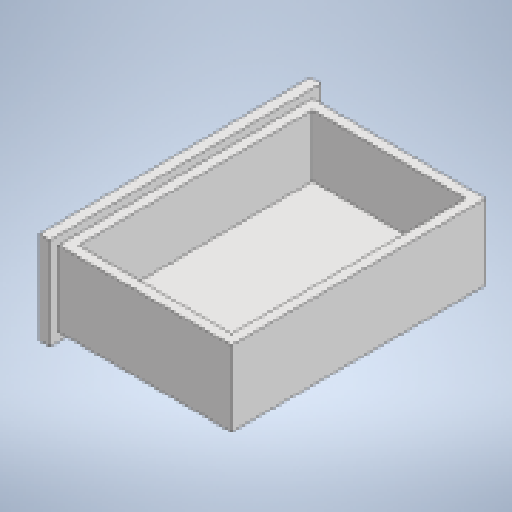
# Autodesk Inventor part: Cajon
Saved by Autodesk Inventor 2024 (Build 280153000, 153)
## iProperties
Created: 2025-02-23
Part Number: Cajon
Material: Genérico
Document SubType Name: Modeling
Designer: sergi
Density: 1 g/cm^3
Appearance: Valor por defecto
Author: sergi
Autodesk Inventor part; units mm, degrees
ref_plane "YZ Plane" through (0, 0, 0) normal (1, 0, 0) x (0, 1, 0)
ref_plane "XZ Plane" through (0, 0, 0) normal (0, 1, 0) x (-1, 0, 0)
ref_plane "XY Plane" through (0, 0, 0) normal (0, 0, 1) x (1, 0, 0)
sketch "Boceto1" plane through (0, 0, 0) normal (0, 1, 0) x (-1, 0, 0)
  line L0 (-121, -177.5) -> (121, -177.5)
  line L1 (121, -177.5) -> (121, 177.5)
  line L2 (121, 177.5) -> (-121, 177.5)
  line L3 (-121, 177.5) -> (-121, -177.5)
  line L4 (-121, -177.5) -> (121, 177.5) construction
  line L5 (121, -177.5) -> (-121, 177.5) construction
  point P0 (0, 0)
  dimension "d0" = 242
  dimension "d1" = 355
  constraints: 12 end point, 2 midpoint, 2 parallel, 1 horizontal, 1 perpendicular
  measures "d0" distance of L2.end L1.end
  measures "d1" distance of L1.end L0.end
extrude "Extrusión1" add sketch "Boceto1" along normal blind 105
sketch "Boceto2" plane through (0, 105, 0) normal (0, 1, 0) x (1, 0, 0)
  line L0 (-121, 177.5) -> (-121, -177.5) projected
  line L1 (-121, -177.5) -> (121, -177.5) projected
  line L2 (121, -177.5) -> (121, 177.5) projected
  line L3 (121, 177.5) -> (-121, 177.5) projected
  line L4 (107, -163.5) -> (-107, -163.5)
  line L5 (-107, -163.5) -> (-107, 163.5)
  line L6 (-107, 163.5) -> (107, 163.5)
  line L7 (107, 163.5) -> (107, -163.5)
  point P0 (0, 0)
  dimension "d4" = 14
  constraints: 8 end point, 3 other
  measures "d4" distance between parallel lines of L1 L4
extrude "Extrusión2" cut sketch "Boceto2" against normal blind 86 contours L4 L5 L6 L7
sketch "Boceto3" plane through (0, 0, 0) normal (0, -1, 0) x (1, 0, 0)
  line L0 (-121, -177.5) -> (-121, 177.5) projected
  line L1 (121, -177.5) -> (-121, -177.5) projected
  line L2 (121, 177.5) -> (121, -177.5) projected
  line L3 (-121, 177.5) -> (121, 177.5) projected
  line L4 (107, 163.5) -> (107, -163.5)
  line L5 (107, -163.5) -> (-107, -163.5)
  line L6 (-107, -163.5) -> (-107, 163.5)
  line L7 (-107, 163.5) -> (107, 163.5)
  point P0 (0, 0)
  dimension "d7" = 14
  constraints: 8 end point, 3 other
  measures "d7" distance between parallel lines of L3 L7
extrude "Extrusión3" cut sketch "Boceto3" against normal blind 16 contours L4 L5 L6 L7
sketch "Boceto4" plane through (-121, 0, -177.5) normal (-1, 0, 0) x (0, 0, 1)
  line L0 (0, 0) -> (355, 0) projected
  line L1 (355, 0) -> (355, 105) projected
  line L2 (0, 105) -> (355, 105) projected
  line L3 (0, 0) -> (0, 105) projected
  line L4 (355, 105) -> (355, 117)
  line L5 (355, 105) -> (367, 105) construction
  line L6 (355, 117) -> (367, 117)
  line L7 (0, 0) -> (-12, 0)
  line L8 (-12, 0) -> (-12, -12)
  line L9 (-12, -12) -> (367, -12)
  line L10 (367, -12) -> (367, 117)
  line L11 (367, 117) -> (-12, 117)
  line L12 (-12, 117) -> (-12, -12)
  point P0 (177.5, 0)
  point P1 (-12, 0)
  dimension "d10" = 12
  dimension "d11" = 90
  dimension "d12" = 12
  dimension "d13" = 90
  dimension "d14" = 12
  dimension "d15" = 12
  dimension "d16" = 90
  constraints: 18 end point, 4 perpendicular, 3 horizontal, 2 parallel, 1 vertical
  measures "d10" distance of L1.end L4.end
  measures "d11" angle of L5 L4
  measures "d12" distance of L4.end L6.end
  measures "d13" angle of L4 L6
  measures "d14" distance of L0.start L7.end
  measures "d15" distance of L7.end L8.end
  measures "d16" angle of L8 L7
extrude "Extrusión4" add sketch "Boceto4" along normal blind 15
sketch "Boceto5" plane through (-136, 0, -177.5) normal (-1, 0, 0) x (0, 0, 1)
  line L0 (-12, 117) -> (-12, -12) projected
  line L1 (-12, -12) -> (367, -12) projected
  line L2 (367, -12) -> (367, 117) projected
  line L3 (367, 117) -> (-12, 117) projected
  line L4 (-12, -12) -> (367, 117)
  circle A0 centre (177.5, 52.5) radius 10
  point P0 (177.5, 0)
  dimension "d19" = 20
  constraints: 2 end point, 1 centre point, 1 midpoint
  measures "d19" diameter of A0
extrude "Extrusión5" add sketch "Boceto5" along normal blind 30 contours A0 L4 | L4 A0
